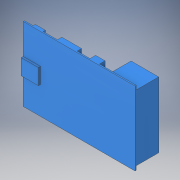
# Autodesk Inventor part: Raspi
Saved by Autodesk Inventor 2019 (Build 230136000, 136)
## iProperties
Created: 2018-12-25
Part Number: Raspi
Material: Generic
Document SubType Name: Modeling
Designer: Martin
Density: 1 g/cm^3
Appearance: Default
Author: Martin
Autodesk Inventor part; units mm, degrees
ref_plane "YZ Plane" through (0, 0, 0) normal (1, 0, 0) x (0, 1, 0)
ref_plane "XZ Plane" through (0, 0, 0) normal (0, 1, 0) x (-1, 0, 0)
ref_plane "XY Plane" through (0, 0, 0) normal (0, 0, 1) x (1, 0, 0)
sketch "Sketch1" plane through (0, 0, 0) normal (0, 0, 1) x (1, 0, 0)
  line L0 (42.5, -28) -> (-42.5, -28)
  line L1 (-42.5, -28) -> (-42.5, 28)
  line L2 (-42.5, 28) -> (42.5, 28)
  line L3 (42.5, 28) -> (42.5, -28)
  line L4 (42.5, -28) -> (-42.5, 28) construction
  line L5 (-42.5, -28) -> (42.5, 28) construction
  point P0 (0, 0)
  dimension "d0" = 85
  dimension "d1" = 56
  constraints: 12 end point, 2 midpoint, 2 parallel, 1 horizontal, 1 perpendicular
  measures "d0" distance of L1.end L2.end
  measures "d1" distance of L0.end L1.end
extrude "Extrusion1" add sketch "Sketch1" along normal blind 1
sketch "Sketch2" plane through (42.5, -28, 0) normal (1, 0, 0) x (0, 0, -1)
  line L0 (0, 56) -> (0, 0) projected
  line L1 (0, 53) -> (17, 53)
  line L2 (17, 53) -> (17, 3)
  line L3 (17, 3) -> (0, 3)
  line L4 (0, 3) -> (0, 53)
  line L5 (0, 56) -> (-1, 56) projected
  line L6 (0, 0) -> (-1, 0) projected
  point P0 (0, 28)
  dimension "d4" = 3
  dimension "d5" = 3
  dimension "d6" = 17
  constraints: 8 end point, 2 parallel, 1 horizontal, 1 perpendicular, 1 point on line
  measures "d4" distance between parallel lines of L1 L5
  measures "d5" distance between parallel lines of L6 L3
  measures "d6" distance of L1.start L1.end
extrude "Extrusion2" add sketch "Sketch2" against normal blind 21
sketch "Sketch3" plane through (-42.5, 28, 0) normal (0, 1, 0) x (1, 0, 0)
  line L0 (49.8, 0) -> (57, 0)
  line L1 (57, 0) -> (57, 4.2398)
  line L2 (57, 4.2398) -> (49.8, 4.2398)
  line L3 (49.8, 4.2398) -> (49.8, 0)
  line L4 (25, 0) -> (40, 0)
  line L5 (40, 0) -> (40, 3.3654)
  line L6 (40, 3.3654) -> (25, 3.3654)
  line L7 (25, 3.3654) -> (25, 0)
  line L8 (6.5, 1.6827) -> (14.1, 1.6827)
  line L9 (14.1, 1.6827) -> (14.1, 0)
  line L10 (14.1, 0) -> (6.5, 0)
  line L11 (6.5, 0) -> (6.5, 1.6827)
  line L12 (85, 0) -> (85, -1) projected
  line L13 (0, 0) -> (0, -1) projected
  point P0 (42.5, 0)
  dimension "d9" = 28
  dimension "d10" = 7.2
  dimension "d11" = 6.5
  dimension "d12" = 7.6
  dimension "d13" = 15
  dimension "d14" = 25
  constraints: 24 end point, 6 parallel, 3 horizontal, 3 perpendicular, 2 point on line
  measures "d9" distance between parallel lines of L12 L1
  measures "d10" distance of L1.end L2.end
  measures "d11" distance between parallel lines of L13 L11
  measures "d12" distance of L8.start L8.end
  measures "d13" distance of L5.end L6.end
  measures "d14" distance between parallel lines of L13 L7
extrude "Extrusion3" add sketch "Sketch3" against normal blind 10
sketch "Sketch4" plane through (0, 0, 1) normal (0, 0, 1) x (1, 0, 0)
  line L0 (-42.5, -7.0526) -> (-29.5, -7.0526)
  line L1 (-29.5, -7.0526) -> (-29.5, 4.9474)
  line L2 (-29.5, 4.9474) -> (-42.5, 4.9474)
  line L3 (-42.5, 4.9474) -> (-42.5, -7.0526)
  line L4 (-42.5, 28) -> (-42.5, -28) projected
  point P0 (0, 0)
  dimension "d17" = 12
  dimension "d18" = 13
  constraints: 8 end point, 2 parallel, 1 collinear, 1 horizontal, 1 perpendicular
  measures "d17" distance of L2.end L0.start
  measures "d18" distance of L1.end L2.end
extrude "Extrusion4" add sketch "Sketch4" along normal blind 1.5
body "Solid1"
